Autodesk Inventor part; units mm, degrees
(part 2 of 2)
sketch "Sketch6" plane through (-21, -26.6, 14.3) normal (0, -1, 0) x (1, 0, 0)
  circle A0 centre (20, -9.6433) radius 3 projected
  arc A1 (9.5506, -10.6725) -> (10.7134, -10.9278) centre (11.3219, -5.3807) ccw projected
  arc A2 (10.7134, -10.9278) -> (10.771, -11.2914) centre (20, -9.6433) ccw projected
  arc A3 (10.771, -11.2914) -> (9.744, -11.8936) centre (13.0638, -16.379) ccw projected
  arc A4 (9.744, -11.8936) -> (9.8402, -12.2945) centre (20, -9.6433) ccw projected
  arc A5 (9.8402, -12.2945) -> (11.0287, -12.3648) centre (10.7619, -6.7907) ccw projected
  arc A6 (11.0287, -12.3648) -> (11.1424, -12.7149) centre (20, -9.6433) ccw projected
  arc A7 (11.1424, -12.7149) -> (10.2222, -13.4703) centre (14.2029, -17.3812) ccw projected
  arc A8 (10.2222, -13.4703) -> (10.38, -13.8512) centre (20, -9.6433) ccw projected
  arc A9 (10.38, -13.8512) -> (11.5649, -13.7347) centre (10.4294, -8.271) ccw projected
  arc A10 (11.5649, -13.7347) -> (11.732, -14.0627) centre (20, -9.6433) ccw projected
  arc A11 (11.732, -14.0627) -> (10.9413, -14.9527) centre (15.4848, -18.1928) ccw projected
  arc A12 (10.9413, -14.9527) -> (11.1567, -15.3043) centre (20, -9.6433) ccw projected
  arc A13 (11.1567, -15.3043) -> (12.3087, -15.0039) centre (10.3325, -9.7851) ccw projected
  arc A14 (12.3087, -15.0039) -> (12.5251, -15.3017) centre (20, -9.6433) ccw projected
  arc A15 (12.5251, -15.3017) -> (11.8834, -16.3045) centre (16.8778, -18.7939) ccw projected
  arc A16 (11.8834, -16.3045) -> (12.1512, -16.618) centre (20, -9.6433) ccw projected
  arc A17 (12.1512, -16.618) -> (13.242, -16.141) centre (10.4737, -11.2957) ccw projected
  arc A18 (13.242, -16.141) -> (13.5023, -16.4013) centre (20, -9.6433) ccw projected
  arc A19 (13.5023, -16.4013) -> (13.0253, -17.4922) centre (18.3477, -19.1696) ccw projected
  arc A20 (13.0253, -17.4922) -> (13.3389, -17.7599) centre (20, -9.6433) ccw projected
  arc A21 (13.3389, -17.7599) -> (14.3417, -17.1182) centre (10.8495, -12.7656) ccw projected
  arc A22 (14.3417, -17.1182) -> (14.6395, -17.3346) centre (20, -9.6433) ccw projected
  arc A23 (14.6395, -17.3346) -> (14.339, -18.4866) centre (19.8582, -19.3108) ccw projected
  arc A24 (14.339, -18.4866) -> (14.6906, -18.7021) centre (20, -9.6433) ccw projected
  arc A25 (14.6906, -18.7021) -> (15.5807, -17.9114) centre (11.4506, -14.1586) ccw projected
  arc A26 (15.5807, -17.9114) -> (15.9087, -18.0785) centre (20, -9.6433) ccw projected
  arc A27 (15.9087, -18.0785) -> (15.7921, -19.2633) centre (21.3723, -19.214) ccw projected
  arc A28 (15.7921, -19.2633) -> (16.1731, -19.4211) centre (20, -9.6433) ccw projected
  arc A29 (16.1731, -19.4211) -> (16.9285, -18.5009) centre (12.2622, -15.4404) ccw projected
  arc A30 (16.9285, -18.5009) -> (17.2786, -18.6147) centre (20, -9.6433) ccw projected
  arc A31 (17.2786, -18.6147) -> (17.3488, -19.8031) centre (22.8526, -18.8815) ccw projected
  arc A32 (17.3488, -19.8031) -> (17.7498, -19.8994) centre (20, -9.6433) ccw projected
  arc A33 (17.7498, -19.8994) -> (18.3519, -18.8723) centre (13.2643, -16.5795) ccw projected
  arc A34 (18.3519, -18.8723) -> (18.7155, -18.9299) centre (20, -9.6433) ccw projected
  arc A35 (18.7155, -18.9299) -> (18.9708, -20.0928) centre (24.2626, -18.3215) ccw projected
  arc A36 (18.9708, -20.0928) -> (19.3819, -20.1251) centre (20, -9.6433) ccw projected
  arc A37 (19.3819, -20.1251) -> (19.8159, -19.0165) centre (14.4323, -17.5478) ccw projected
  arc A38 (19.8159, -19.0165) -> (20.1841, -19.0165) centre (20, -9.6433) ccw projected
  arc A39 (20.1841, -19.0165) -> (20.6181, -20.1251) centre (25.5677, -17.5478) ccw projected
  arc A40 (20.6181, -20.1251) -> (21.0292, -20.0928) centre (20, -9.6433) ccw projected
  arc A41 (21.0292, -20.0928) -> (21.2845, -18.9299) centre (15.7374, -18.3215) ccw projected
  arc A42 (21.2845, -18.9299) -> (21.6481, -18.8723) centre (20, -9.6433) ccw projected
  arc A43 (21.6481, -18.8723) -> (22.2502, -19.8994) centre (26.7357, -16.5795) ccw projected
  arc A44 (22.2502, -19.8994) -> (22.6512, -19.8031) centre (20, -9.6433) ccw projected
  arc A45 (22.6512, -19.8031) -> (22.7214, -18.6147) centre (17.1474, -18.8815) ccw projected
  arc A46 (22.7214, -18.6147) -> (23.0715, -18.5009) centre (20, -9.6433) ccw projected
  arc A47 (23.0715, -18.5009) -> (23.8269, -19.4211) centre (27.7378, -15.4404) ccw projected
  arc A48 (23.8269, -19.4211) -> (24.2079, -19.2633) centre (20, -9.6433) ccw projected
  arc A49 (24.2079, -19.2633) -> (24.0913, -18.0785) centre (18.6277, -19.214) ccw projected
  arc A50 (24.0913, -18.0785) -> (24.4193, -17.9114) centre (20, -9.6433) ccw projected
  arc A51 (24.4193, -17.9114) -> (25.3094, -18.7021) centre (28.5494, -14.1586) ccw projected
  arc A52 (25.3094, -18.7021) -> (25.661, -18.4866) centre (20, -9.6433) ccw projected
  arc A53 (25.661, -18.4866) -> (25.3605, -17.3346) centre (20.1418, -19.3108) ccw projected
  arc A54 (25.3605, -17.3346) -> (25.6583, -17.1182) centre (20, -9.6433) ccw projected
  arc A55 (25.6583, -17.1182) -> (26.6611, -17.7599) centre (29.1505, -12.7656) ccw projected
  arc A56 (26.6611, -17.7599) -> (26.9747, -17.4922) centre (20, -9.6433) ccw projected
  arc A57 (26.9747, -17.4922) -> (26.4977, -16.4013) centre (21.6523, -19.1696) ccw projected
  arc A58 (26.4977, -16.4013) -> (26.758, -16.141) centre (20, -9.6433) ccw projected
  arc A59 (26.758, -16.141) -> (27.8488, -16.618) centre (29.5263, -11.2957) ccw projected
  arc A60 (27.8488, -16.618) -> (28.1166, -16.3045) centre (20, -9.6433) ccw projected
  arc A61 (28.1166, -16.3045) -> (27.4749, -15.3017) centre (23.1222, -18.7939) ccw projected
  arc A62 (27.4749, -15.3017) -> (27.6913, -15.0039) centre (20, -9.6433) ccw projected
  arc A63 (27.6913, -15.0039) -> (28.8433, -15.3043) centre (29.6675, -9.7851) ccw projected
  arc A64 (28.8433, -15.3043) -> (29.0587, -14.9527) centre (20, -9.6433) ccw projected
  arc A65 (29.0587, -14.9527) -> (28.268, -14.0627) centre (24.5152, -18.1928) ccw projected
  arc A66 (28.268, -14.0627) -> (28.4351, -13.7347) centre (20, -9.6433) ccw projected
  arc A67 (28.4351, -13.7347) -> (29.62, -13.8512) centre (29.5706, -8.271) ccw projected
  arc A68 (29.62, -13.8512) -> (29.7778, -13.4703) centre (20, -9.6433) ccw projected
  arc A69 (29.7778, -13.4703) -> (28.8576, -12.7149) centre (25.7971, -17.3812) ccw projected
  arc A70 (28.8576, -12.7149) -> (28.9713, -12.3648) centre (20, -9.6433) ccw projected
  arc A71 (28.9713, -12.3648) -> (30.1598, -12.2945) centre (29.2381, -6.7907) ccw projected
  arc A72 (30.1598, -12.2945) -> (30.256, -11.8936) centre (20, -9.6433) ccw projected
  arc A73 (30.256, -11.8936) -> (29.229, -11.2914) centre (26.9362, -16.379) ccw projected
  arc A74 (29.229, -11.2914) -> (29.2866, -10.9278) centre (20, -9.6433) ccw projected
  arc A75 (29.2866, -10.9278) -> (30.4494, -10.6725) centre (28.6781, -5.3807) ccw projected
  arc A76 (30.4494, -10.6725) -> (30.4818, -10.2615) centre (20, -9.6433) ccw projected
  arc A77 (30.4818, -10.2615) -> (29.3732, -9.8274) centre (27.9045, -15.2111) ccw projected
  arc A78 (29.3732, -9.8274) -> (29.3732, -9.4593) centre (20, -9.6433) ccw projected
  arc A79 (29.3732, -9.4593) -> (30.4818, -9.0252) centre (27.9045, -4.0756) ccw projected
  arc A80 (30.4818, -9.0252) -> (30.4494, -8.6142) centre (20, -9.6433) ccw projected
  arc A81 (30.4494, -8.6142) -> (29.2866, -8.3588) centre (28.6781, -13.906) ccw projected
  arc A82 (29.2866, -8.3588) -> (29.229, -7.9952) centre (20, -9.6433) ccw projected
  arc A83 (29.229, -7.9952) -> (30.256, -7.3931) centre (26.9362, -2.9076) ccw projected
  arc A84 (30.256, -7.3931) -> (30.1598, -6.9922) centre (20, -9.6433) ccw projected
  arc A85 (30.1598, -6.9922) -> (28.9713, -6.9219) centre (29.2381, -12.4959) ccw projected
  arc A86 (28.9713, -6.9219) -> (28.8576, -6.5718) centre (20, -9.6433) ccw projected
  arc A87 (28.8576, -6.5718) -> (29.7778, -5.8164) centre (25.7971, -1.9055) ccw projected
  arc A88 (29.7778, -5.8164) -> (29.62, -5.4355) centre (20, -9.6433) ccw projected
  arc A89 (29.62, -5.4355) -> (28.4351, -5.552) centre (29.5706, -11.0157) ccw projected
  arc A90 (28.4351, -5.552) -> (28.268, -5.224) centre (20, -9.6433) ccw projected
  arc A91 (28.268, -5.224) -> (29.0587, -4.3339) centre (24.5152, -1.0939) ccw projected
  arc A92 (29.0587, -4.3339) -> (28.8433, -3.9824) centre (20, -9.6433) ccw projected
  arc A93 (28.8433, -3.9824) -> (27.6913, -4.2828) centre (29.6675, -9.5016) ccw projected
  arc A94 (27.6913, -4.2828) -> (27.4749, -3.985) centre (20, -9.6433) ccw projected
  arc A95 (27.4749, -3.985) -> (28.1166, -2.9822) centre (23.1222, -0.4928) ccw projected
  arc A96 (28.1166, -2.9822) -> (27.8488, -2.6687) centre (20, -9.6433) ccw projected
  arc A97 (27.8488, -2.6687) -> (26.758, -3.1456) centre (29.5263, -7.991) ccw projected
  arc A98 (26.758, -3.1456) -> (26.4977, -2.8853) centre (20, -9.6433) ccw projected
  arc A99 (26.4977, -2.8853) -> (26.9747, -1.7945) centre (21.6523, -0.1171) ccw projected
  arc A100 (26.9747, -1.7945) -> (26.6611, -1.5267) centre (20, -9.6433) ccw projected
  arc A101 (26.6611, -1.5267) -> (25.6583, -2.1685) centre (29.1505, -6.5211) ccw projected
  arc A102 (25.6583, -2.1685) -> (25.3605, -1.9521) centre (20, -9.6433) ccw projected
  arc A103 (25.3605, -1.9521) -> (25.661, -0.8001) centre (20.1418, 0.0241) ccw projected
  arc A104 (25.661, -0.8001) -> (25.3094, -0.5846) centre (20, -9.6433) ccw projected
  arc A105 (25.3094, -0.5846) -> (24.4193, -1.3753) centre (28.5494, -5.1281) ccw projected
  arc A106 (24.4193, -1.3753) -> (24.0913, -1.2082) centre (20, -9.6433) ccw projected
  arc A107 (24.0913, -1.2082) -> (24.2079, -0.0234) centre (18.6277, -0.0727) ccw projected
  arc A108 (24.2079, -0.0234) -> (23.8269, 0.1344) centre (20, -9.6433) ccw projected
  arc A109 (23.8269, 0.1344) -> (23.0715, -0.7858) centre (27.7378, -3.8463) ccw projected
  arc A110 (23.0715, -0.7858) -> (22.7214, -0.672) centre (20, -9.6433) ccw projected
  arc A111 (22.7214, -0.672) -> (22.6512, 0.5165) centre (17.1474, -0.4052) ccw projected
  arc A112 (22.6512, 0.5165) -> (22.2502, 0.6127) centre (20, -9.6433) ccw projected
  arc A113 (22.2502, 0.6127) -> (21.6481, -0.4143) centre (26.7357, -2.7072) ccw projected
  arc A114 (21.6481, -0.4143) -> (21.2845, -0.3568) centre (20, -9.6433) ccw projected
  arc A115 (21.2845, -0.3568) -> (21.0292, 0.8061) centre (15.7374, -0.9652) ccw projected
  arc A116 (21.0292, 0.8061) -> (20.6181, 0.8384) centre (20, -9.6433) ccw projected
  arc A117 (20.6181, 0.8384) -> (20.1841, -0.2701) centre (25.5677, -1.7389) ccw projected
  arc A118 (20.1841, -0.2701) -> (19.8159, -0.2701) centre (20, -9.6433) ccw projected
  arc A119 (19.8159, -0.2701) -> (19.3819, 0.8384) centre (14.4323, -1.7389) ccw projected
  arc A120 (19.3819, 0.8384) -> (18.9708, 0.8061) centre (20, -9.6433) ccw projected
  arc A121 (18.9708, 0.8061) -> (18.7155, -0.3568) centre (24.2626, -0.9652) ccw projected
  arc A122 (18.7155, -0.3568) -> (18.3519, -0.4143) centre (20, -9.6433) ccw projected
  arc A123 (18.3519, -0.4143) -> (17.7498, 0.6127) centre (13.2643, -2.7072) ccw projected
  arc A124 (17.7498, 0.6127) -> (17.3488, 0.5165) centre (20, -9.6433) ccw projected
  arc A125 (17.3488, 0.5165) -> (17.2786, -0.672) centre (22.8526, -0.4052) ccw projected
  arc A126 (17.2786, -0.672) -> (16.9285, -0.7858) centre (20, -9.6433) ccw projected
  arc A127 (16.9285, -0.7858) -> (16.1731, 0.1344) centre (12.2622, -3.8463) ccw projected
  arc A128 (16.1731, 0.1344) -> (15.7921, -0.0234) centre (20, -9.6433) ccw projected
  arc A129 (15.7921, -0.0234) -> (15.9087, -1.2082) centre (21.3723, -0.0727) ccw projected
  arc A130 (15.9087, -1.2082) -> (15.5807, -1.3753) centre (20, -9.6433) ccw projected
  arc A131 (15.5807, -1.3753) -> (14.6906, -0.5846) centre (11.4506, -5.1281) ccw projected
  arc A132 (14.6906, -0.5846) -> (14.339, -0.8001) centre (20, -9.6433) ccw projected
  arc A133 (14.339, -0.8001) -> (14.6395, -1.9521) centre (19.8582, 0.0241) ccw projected
  arc A134 (14.6395, -1.9521) -> (14.3417, -2.1685) centre (20, -9.6433) ccw projected
  arc A135 (14.3417, -2.1685) -> (13.3389, -1.5267) centre (10.8495, -6.5211) ccw projected
  arc A136 (13.3389, -1.5267) -> (13.0253, -1.7945) centre (20, -9.6433) ccw projected
  arc A137 (13.0253, -1.7945) -> (13.5023, -2.8853) centre (18.3477, -0.1171) ccw projected
  arc A138 (13.5023, -2.8853) -> (13.242, -3.1456) centre (20, -9.6433) ccw projected
  arc A139 (13.242, -3.1456) -> (12.1512, -2.6687) centre (10.4737, -7.991) ccw projected
  arc A140 (12.1512, -2.6687) -> (11.8834, -2.9822) centre (20, -9.6433) ccw projected
  arc A141 (11.8834, -2.9822) -> (12.5251, -3.985) centre (16.8778, -0.4928) ccw projected
  arc A142 (12.5251, -3.985) -> (12.3087, -4.2828) centre (20, -9.6433) ccw projected
  arc A143 (12.3087, -4.2828) -> (11.1567, -3.9824) centre (10.3325, -9.5016) ccw projected
  arc A144 (11.1567, -3.9824) -> (10.9413, -4.3339) centre (20, -9.6433) ccw projected
  arc A145 (10.9413, -4.3339) -> (11.732, -5.224) centre (15.4848, -1.0939) ccw projected
  arc A146 (11.732, -5.224) -> (11.5649, -5.552) centre (20, -9.6433) ccw projected
  arc A147 (11.5649, -5.552) -> (10.38, -5.4355) centre (10.4294, -11.0157) ccw projected
  arc A148 (10.38, -5.4355) -> (10.2222, -5.8164) centre (20, -9.6433) ccw projected
  arc A149 (10.2222, -5.8164) -> (11.1424, -6.5718) centre (14.2029, -1.9055) ccw projected
  arc A150 (11.1424, -6.5718) -> (11.0287, -6.9219) centre (20, -9.6433) ccw projected
  arc A151 (11.0287, -6.9219) -> (9.8402, -6.9922) centre (10.7619, -12.4959) ccw projected
  arc A152 (9.8402, -6.9922) -> (9.744, -7.3931) centre (20, -9.6433) ccw projected
  arc A153 (9.744, -7.3931) -> (10.771, -7.9952) centre (13.0638, -2.9076) ccw projected
  arc A154 (10.771, -7.9952) -> (10.7134, -8.3588) centre (20, -9.6433) ccw projected
  arc A155 (10.7134, -8.3588) -> (9.5506, -8.6142) centre (11.3219, -13.906) ccw projected
  arc A156 (9.5506, -8.6142) -> (9.5182, -9.0252) centre (20, -9.6433) ccw projected
  arc A157 (9.5182, -9.0252) -> (10.6268, -9.4593) centre (12.0955, -4.0756) ccw projected
  arc A158 (10.6268, -9.4593) -> (10.6268, -9.8274) centre (20, -9.6433) ccw projected
  arc A159 (10.6268, -9.8274) -> (9.5182, -10.2615) centre (12.0955, -15.2111) ccw projected
  arc A160 (9.5182, -10.2615) -> (9.5506, -10.6725) centre (20, -9.6433) ccw projected
  circle A161 centre (47, -9.6433) radius 3 projected
  arc A162 (57.4494, -8.6142) -> (56.2866, -8.3588) centre (55.6781, -13.906) ccw projected
  arc A163 (56.2866, -8.3588) -> (56.229, -7.9952) centre (47, -9.6433) ccw projected
  arc A164 (56.229, -7.9952) -> (57.256, -7.3931) centre (53.9362, -2.9076) ccw projected
  arc A165 (57.256, -7.3931) -> (57.1598, -6.9922) centre (47, -9.6433) ccw projected
  arc A166 (57.1598, -6.9922) -> (55.9713, -6.9219) centre (56.2381, -12.4959) ccw projected
  arc A167 (55.9713, -6.9219) -> (55.8576, -6.5718) centre (47, -9.6433) ccw projected
  arc A168 (55.8576, -6.5718) -> (56.7778, -5.8164) centre (52.7971, -1.9055) ccw projected
  arc A169 (56.7778, -5.8164) -> (56.62, -5.4355) centre (47, -9.6433) ccw projected
  arc A170 (56.62, -5.4355) -> (55.4351, -5.552) centre (56.5706, -11.0157) ccw projected
  arc A171 (55.4351, -5.552) -> (55.268, -5.224) centre (47, -9.6433) ccw projected
  arc A172 (55.268, -5.224) -> (56.0587, -4.3339) centre (51.5152, -1.0939) ccw projected
  arc A173 (56.0587, -4.3339) -> (55.8433, -3.9824) centre (47, -9.6433) ccw projected
  arc A174 (55.8433, -3.9824) -> (54.6913, -4.2828) centre (56.6675, -9.5016) ccw projected
  arc A175 (54.6913, -4.2828) -> (54.4749, -3.985) centre (47, -9.6433) ccw projected
  arc A176 (54.4749, -3.985) -> (55.1166, -2.9822) centre (50.1222, -0.4928) ccw projected
  arc A177 (55.1166, -2.9822) -> (54.8488, -2.6687) centre (47, -9.6433) ccw projected
  arc A178 (54.8488, -2.6687) -> (53.758, -3.1456) centre (56.5263, -7.991) ccw projected
  arc A179 (53.758, -3.1456) -> (53.4977, -2.8853) centre (47, -9.6433) ccw projected
  arc A180 (53.4977, -2.8853) -> (53.9747, -1.7945) centre (48.6523, -0.1171) ccw projected
  arc A181 (53.9747, -1.7945) -> (53.6611, -1.5267) centre (47, -9.6433) ccw projected
  arc A182 (53.6611, -1.5267) -> (52.6583, -2.1685) centre (56.1505, -6.5211) ccw projected
  arc A183 (52.6583, -2.1685) -> (52.3605, -1.9521) centre (47, -9.6433) ccw projected
  arc A184 (52.3605, -1.9521) -> (52.661, -0.8001) centre (47.1418, 0.0241) ccw projected
  arc A185 (52.661, -0.8001) -> (52.3094, -0.5846) centre (47, -9.6433) ccw projected
  arc A186 (52.3094, -0.5846) -> (51.4193, -1.3753) centre (55.5494, -5.1281) ccw projected
  arc A187 (51.4193, -1.3753) -> (51.0913, -1.2082) centre (47, -9.6433) ccw projected
  arc A188 (51.0913, -1.2082) -> (51.2079, -0.0234) centre (45.6277, -0.0727) ccw projected
  arc A189 (51.2079, -0.0234) -> (50.8269, 0.1344) centre (47, -9.6433) ccw projected
  arc A190 (50.8269, 0.1344) -> (50.0715, -0.7858) centre (54.7378, -3.8463) ccw projected
  arc A191 (50.0715, -0.7858) -> (49.7214, -0.672) centre (47, -9.6433) ccw projected
  arc A192 (49.7214, -0.672) -> (49.6512, 0.5165) centre (44.1474, -0.4052) ccw projected
  arc A193 (49.6512, 0.5165) -> (49.2502, 0.6127) centre (47, -9.6433) ccw projected
  arc A194 (49.2502, 0.6127) -> (48.6481, -0.4143) centre (53.7357, -2.7072) ccw projected
  arc A195 (48.6481, -0.4143) -> (48.2845, -0.3568) centre (47, -9.6433) ccw projected
  arc A196 (48.2845, -0.3568) -> (48.0292, 0.8061) centre (42.7374, -0.9652) ccw projected
  arc A197 (48.0292, 0.8061) -> (47.6181, 0.8384) centre (47, -9.6433) ccw projected
  arc A198 (47.6181, 0.8384) -> (47.1841, -0.2701) centre (52.5677, -1.7389) ccw projected
  arc A199 (47.1841, -0.2701) -> (46.8159, -0.2701) centre (47, -9.6433) ccw projected
  arc A200 (46.8159, -0.2701) -> (46.3819, 0.8384) centre (41.4323, -1.7389) ccw projected
  arc A201 (46.3819, 0.8384) -> (45.9708, 0.8061) centre (47, -9.6433) ccw projected
  arc A202 (45.9708, 0.8061) -> (45.7155, -0.3568) centre (51.2626, -0.9652) ccw projected
  arc A203 (45.7155, -0.3568) -> (45.3519, -0.4143) centre (47, -9.6433) ccw projected
  arc A204 (45.3519, -0.4143) -> (44.7498, 0.6127) centre (40.2643, -2.7072) ccw projected
  arc A205 (44.7498, 0.6127) -> (44.3488, 0.5165) centre (47, -9.6433) ccw projected
  arc A206 (44.3488, 0.5165) -> (44.2786, -0.672) centre (49.8526, -0.4052) ccw projected
  arc A207 (44.2786, -0.672) -> (43.9285, -0.7858) centre (47, -9.6433) ccw projected
  arc A208 (43.9285, -0.7858) -> (43.1731, 0.1344) centre (39.2622, -3.8463) ccw projected
  arc A209 (43.1731, 0.1344) -> (42.7921, -0.0234) centre (47, -9.6433) ccw projected
  arc A210 (42.7921, -0.0234) -> (42.9087, -1.2082) centre (48.3723, -0.0727) ccw projected
  arc A211 (42.9087, -1.2082) -> (42.5807, -1.3753) centre (47, -9.6433) ccw projected
  arc A212 (42.5807, -1.3753) -> (41.6906, -0.5846) centre (38.4506, -5.1281) ccw projected
  arc A213 (41.6906, -0.5846) -> (41.339, -0.8001) centre (47, -9.6433) ccw projected
  arc A214 (41.339, -0.8001) -> (41.6395, -1.9521) centre (46.8582, 0.0241) ccw projected
  arc A215 (41.6395, -1.9521) -> (41.3417, -2.1685) centre (47, -9.6433) ccw projected
  arc A216 (41.3417, -2.1685) -> (40.3389, -1.5267) centre (37.8495, -6.5211) ccw projected
  arc A217 (40.3389, -1.5267) -> (40.0253, -1.7945) centre (47, -9.6433) ccw projected
  arc A218 (40.0253, -1.7945) -> (40.5023, -2.8853) centre (45.3477, -0.1171) ccw projected
  arc A219 (40.5023, -2.8853) -> (40.242, -3.1456) centre (47, -9.6433) ccw projected
  arc A220 (40.242, -3.1456) -> (39.1512, -2.6687) centre (37.4737, -7.991) ccw projected
  arc A221 (39.1512, -2.6687) -> (38.8834, -2.9822) centre (47, -9.6433) ccw projected
  arc A222 (38.8834, -2.9822) -> (39.5251, -3.985) centre (43.8778, -0.4928) ccw projected
  arc A223 (39.5251, -3.985) -> (39.3087, -4.2828) centre (47, -9.6433) ccw projected
  arc A224 (39.3087, -4.2828) -> (38.1567, -3.9824) centre (37.3325, -9.5016) ccw projected
  arc A225 (38.1567, -3.9824) -> (37.9413, -4.3339) centre (47, -9.6433) ccw projected
  arc A226 (37.9413, -4.3339) -> (38.732, -5.224) centre (42.4848, -1.0939) ccw projected
  arc A227 (38.732, -5.224) -> (38.5649, -5.552) centre (47, -9.6433) ccw projected
  arc A228 (38.5649, -5.552) -> (37.38, -5.4355) centre (37.4294, -11.0157) ccw projected
  arc A229 (37.38, -5.4355) -> (37.2222, -5.8164) centre (47, -9.6433) ccw projected
  arc A230 (37.2222, -5.8164) -> (38.1424, -6.5718) centre (41.2029, -1.9055) ccw projected
  arc A231 (38.1424, -6.5718) -> (38.0287, -6.9219) centre (47, -9.6433) ccw projected
  arc A232 (38.0287, -6.9219) -> (36.8402, -6.9922) centre (37.7619, -12.4959) ccw projected
  arc A233 (36.8402, -6.9922) -> (36.744, -7.3931) centre (47, -9.6433) ccw projected
  arc A234 (36.744, -7.3931) -> (37.771, -7.9952) centre (40.0638, -2.9076) ccw projected
  arc A235 (37.771, -7.9952) -> (37.7134, -8.3588) centre (47, -9.6433) ccw projected
  arc A236 (37.7134, -8.3588) -> (36.5506, -8.6142) centre (38.3219, -13.906) ccw projected
  arc A237 (36.5506, -8.6142) -> (36.5182, -9.0252) centre (47, -9.6433) ccw projected
  arc A238 (36.5182, -9.0252) -> (37.6268, -9.4593) centre (39.0955, -4.0756) ccw projected
  arc A239 (37.6268, -9.4593) -> (37.6268, -9.8274) centre (47, -9.6433) ccw projected
  arc A240 (37.6268, -9.8274) -> (36.5182, -10.2615) centre (39.0955, -15.2111) ccw projected
  arc A241 (36.5182, -10.2615) -> (36.5506, -10.6725) centre (47, -9.6433) ccw projected
  arc A242 (36.5506, -10.6725) -> (37.7134, -10.9278) centre (38.3219, -5.3807) ccw projected
  arc A243 (37.7134, -10.9278) -> (37.771, -11.2914) centre (47, -9.6433) ccw projected
  arc A244 (37.771, -11.2914) -> (36.744, -11.8936) centre (40.0638, -16.379) ccw projected
  arc A245 (36.744, -11.8936) -> (36.8402, -12.2945) centre (47, -9.6433) ccw projected
  arc A246 (36.8402, -12.2945) -> (38.0287, -12.3648) centre (37.7619, -6.7907) ccw projected
  arc A247 (38.0287, -12.3648) -> (38.1424, -12.7149) centre (47, -9.6433) ccw projected
  arc A248 (38.1424, -12.7149) -> (37.2222, -13.4703) centre (41.2029, -17.3812) ccw projected
  arc A249 (37.2222, -13.4703) -> (37.38, -13.8512) centre (47, -9.6433) ccw projected
  arc A250 (37.38, -13.8512) -> (38.5649, -13.7347) centre (37.4294, -8.271) ccw projected
  arc A251 (38.5649, -13.7347) -> (38.732, -14.0627) centre (47, -9.6433) ccw projected
  arc A252 (38.732, -14.0627) -> (37.9413, -14.9527) centre (42.4848, -18.1928) ccw projected
  arc A253 (37.9413, -14.9527) -> (38.1567, -15.3043) centre (47, -9.6433) ccw projected
  arc A254 (38.1567, -15.3043) -> (39.3087, -15.0039) centre (37.3325, -9.7851) ccw projected
  arc A255 (39.3087, -15.0039) -> (39.5251, -15.3017) centre (47, -9.6433) ccw projected
  arc A256 (39.5251, -15.3017) -> (38.8834, -16.3045) centre (43.8778, -18.7939) ccw projected
  arc A257 (38.8834, -16.3045) -> (39.1512, -16.618) centre (47, -9.6433) ccw projected
  arc A258 (39.1512, -16.618) -> (40.242, -16.141) centre (37.4737, -11.2957) ccw projected
  arc A259 (40.242, -16.141) -> (40.5023, -16.4013) centre (47, -9.6433) ccw projected
  arc A260 (40.5023, -16.4013) -> (40.0253, -17.4922) centre (45.3477, -19.1696) ccw projected
  arc A261 (40.0253, -17.4922) -> (40.3389, -17.7599) centre (47, -9.6433) ccw projected
  arc A262 (40.3389, -17.7599) -> (41.3417, -17.1182) centre (37.8495, -12.7656) ccw projected
  arc A263 (41.3417, -17.1182) -> (41.6395, -17.3346) centre (47, -9.6433) ccw projected
  arc A264 (41.6395, -17.3346) -> (41.339, -18.4866) centre (46.8582, -19.3108) ccw projected
  arc A265 (41.339, -18.4866) -> (41.6906, -18.7021) centre (47, -9.6433) ccw projected
  arc A266 (41.6906, -18.7021) -> (42.5807, -17.9114) centre (38.4506, -14.1586) ccw projected
  arc A267 (42.5807, -17.9114) -> (42.9087, -18.0785) centre (47, -9.6433) ccw projected
  arc A268 (42.9087, -18.0785) -> (42.7921, -19.2633) centre (48.3723, -19.214) ccw projected
  arc A269 (42.7921, -19.2633) -> (43.1731, -19.4211) centre (47, -9.6433) ccw projected
  arc A270 (43.1731, -19.4211) -> (43.9285, -18.5009) centre (39.2622, -15.4404) ccw projected
  arc A271 (43.9285, -18.5009) -> (44.2786, -18.6147) centre (47, -9.6433) ccw projected
  arc A272 (44.2786, -18.6147) -> (44.3488, -19.8031) centre (49.8526, -18.8815) ccw projected
  arc A273 (44.3488, -19.8031) -> (44.7498, -19.8994) centre (47, -9.6433) ccw projected
  arc A274 (44.7498, -19.8994) -> (45.3519, -18.8723) centre (40.2643, -16.5795) ccw projected
  arc A275 (45.3519, -18.8723) -> (45.7155, -18.9299) centre (47, -9.6433) ccw projected
  arc A276 (45.7155, -18.9299) -> (45.9708, -20.0928) centre (51.2626, -18.3215) ccw projected
  arc A277 (45.9708, -20.0928) -> (46.3819, -20.1251) centre (47, -9.6433) ccw projected
  arc A278 (46.3819, -20.1251) -> (46.8159, -19.0165) centre (41.4323, -17.5478) ccw projected
  arc A279 (46.8159, -19.0165) -> (47.1841, -19.0165) centre (47, -9.6433) ccw projected
  arc A280 (47.1841, -19.0165) -> (47.6181, -20.1251) centre (52.5677, -17.5478) ccw projected
  arc A281 (47.6181, -20.1251) -> (48.0292, -20.0928) centre (47, -9.6433) ccw projected
  arc A282 (48.0292, -20.0928) -> (48.2845, -18.9299) centre (42.7374, -18.3215) ccw projected
  arc A283 (48.2845, -18.9299) -> (48.6481, -18.8723) centre (47, -9.6433) ccw projected
  arc A284 (48.6481, -18.8723) -> (49.2502, -19.8994) centre (53.7357, -16.5795) ccw projected
  arc A285 (49.2502, -19.8994) -> (49.6512, -19.8031) centre (47, -9.6433) ccw projected
  arc A286 (49.6512, -19.8031) -> (49.7214, -18.6147) centre (44.1474, -18.8815) ccw projected
  arc A287 (49.7214, -18.6147) -> (50.0715, -18.5009) centre (47, -9.6433) ccw projected
  arc A288 (50.0715, -18.5009) -> (50.8269, -19.4211) centre (54.7378, -15.4404) ccw projected
  arc A289 (50.8269, -19.4211) -> (51.2079, -19.2633) centre (47, -9.6433) ccw projected
  arc A290 (51.2079, -19.2633) -> (51.0913, -18.0785) centre (45.6277, -19.214) ccw projected
  arc A291 (51.0913, -18.0785) -> (51.4193, -17.9114) centre (47, -9.6433) ccw projected
  arc A292 (51.4193, -17.9114) -> (52.3094, -18.7021) centre (55.5494, -14.1586) ccw projected
  arc A293 (52.3094, -18.7021) -> (52.661, -18.4866) centre (47, -9.6433) ccw projected
  arc A294 (52.661, -18.4866) -> (52.3605, -17.3346) centre (47.1418, -19.3108) ccw projected
  arc A295 (52.3605, -17.3346) -> (52.6583, -17.1182) centre (47, -9.6433) ccw projected
  arc A296 (52.6583, -17.1182) -> (53.6611, -17.7599) centre (56.1505, -12.7656) ccw projected
  arc A297 (53.6611, -17.7599) -> (53.9747, -17.4922) centre (47, -9.6433) ccw projected
  arc A298 (53.9747, -17.4922) -> (53.4977, -16.4013) centre (48.6523, -19.1696) ccw projected
  arc A299 (53.4977, -16.4013) -> (53.758, -16.141) centre (47, -9.6433) ccw projected
  arc A300 (53.758, -16.141) -> (54.8488, -16.618) centre (56.5263, -11.2957) ccw projected
  arc A301 (54.8488, -16.618) -> (55.1166, -16.3045) centre (47, -9.6433) ccw projected
  arc A302 (55.1166, -16.3045) -> (54.4749, -15.3017) centre (50.1222, -18.7939) ccw projected
  arc A303 (54.4749, -15.3017) -> (54.6913, -15.0039) centre (47, -9.6433) ccw projected
  arc A304 (54.6913, -15.0039) -> (55.8433, -15.3043) centre (56.6675, -9.7851) ccw projected
  arc A305 (55.8433, -15.3043) -> (56.0587, -14.9527) centre (47, -9.6433) ccw projected
  arc A306 (56.0587, -14.9527) -> (55.268, -14.0627) centre (51.5152, -18.1928) ccw projected
  arc A307 (55.268, -14.0627) -> (55.4351, -13.7347) centre (47, -9.6433) ccw projected
  arc A308 (55.4351, -13.7347) -> (56.62, -13.8512) centre (56.5706, -8.271) ccw projected
  arc A309 (56.62, -13.8512) -> (56.7778, -13.4703) centre (47, -9.6433) ccw projected
  arc A310 (56.7778, -13.4703) -> (55.8576, -12.7149) centre (52.7971, -17.3812) ccw projected
  arc A311 (55.8576, -12.7149) -> (55.9713, -12.3648) centre (47, -9.6433) ccw projected
  arc A312 (55.9713, -12.3648) -> (57.1598, -12.2945) centre (56.2381, -6.7907) ccw projected
  arc A313 (57.1598, -12.2945) -> (57.256, -11.8936) centre (47, -9.6433) ccw projected
  arc A314 (57.256, -11.8936) -> (56.229, -11.2914) centre (53.9362, -16.379) ccw projected
  arc A315 (56.229, -11.2914) -> (56.2866, -10.9278) centre (47, -9.6433) ccw projected
  arc A316 (56.2866, -10.9278) -> (57.4494, -10.6725) centre (55.6781, -5.3807) ccw projected
  arc A317 (57.4494, -10.6725) -> (57.4818, -10.2615) centre (47, -9.6433) ccw projected
  arc A318 (57.4818, -10.2615) -> (56.3732, -9.8274) centre (54.9045, -15.2111) ccw projected
  arc A319 (56.3732, -9.8274) -> (56.3732, -9.4593) centre (47, -9.6433) ccw projected
  arc A320 (56.3732, -9.4593) -> (57.4818, -9.0252) centre (54.9045, -4.0756) ccw projected
  arc A321 (57.4818, -9.0252) -> (57.4494, -8.6142) centre (47, -9.6433) ccw projected
  circle A322 centre (20, -9.6433) radius 10.5
  circle A323 centre (47, -9.6433) radius 10.5
  circle A324 centre (20, -9.6433) radius 10.9
  circle A325 centre (47, -9.6433) radius 10.9
  arc A326 (29.092, 0.1172) -> (29.2864, -14.3) centre (33.5, -7.0333) ccw projected
  line L0 (6.5, -14.3) -> (29.2864, -14.3) projected
  arc A327 (36.2919, 9.8389) -> (29.092, 0.1172) centre (35.7557, 2.709) ccw projected
  arc A328 (49.3884, 4.2041) -> (36.2919, 9.8389) centre (43.0585, 7.5289) ccw projected
  arc A329 (41.3938, -1.688) -> (49.3884, 4.2041) centre (46.65, -0.45) ccw projected
  arc A330 (40.6022, -2.5478) -> (41.3938, -1.688) centre (35.7557, 2.709) ccw projected
  arc A331 (37.7136, -14.3) -> (40.6022, -2.5478) centre (33.5, -7.0333) ccw projected
  line L1 (37.7136, -14.3) -> (60.5, -14.3) projected
  line L2 (60.5, -14.3) -> (60.5, 13.4) projected
  line L3 (60.5, 13.4) -> (48.1174, 13.4) projected
  arc A332 (48.1174, 13.4) -> (37.9995, 13.4) centre (43.0585, 7.5289) ccw projected
  line L4 (37.9995, 13.4) -> (6.5, 13.4) projected
  line L5 (6.5, 13.4) -> (6.5, -14.3) projected
  point P0 (21, -14.3)
  point P1 (27.2086, -1.4674)
  point P2 (37.2633, -14.5431)
  point P3 (52.0289, 0.0273)
  point P4 (56.8552, -14.3)
  point P5 (10.1448, -14.3)
  dimension "d29" = 0.4
  dimension "d30" = 0.4
  constraints: 2 centre point, 2 coincident, 6 other
ref_plane "Work Plane4" through (-12.2915, -29.7, -6.6348) normal (0, -1, 0) x (0.9969173, 0, -0.0784591)
extrude "Extrusion6" add sketch "Sketch6" along normal blind 3.2 contours L0 L5 L4 A332 L3 L2 L1 A325 A329 A328 A327 A326 A324
sketch "Sketch7" plane through (-21, -26.6, 14.3) normal (0, -1, 0) x (1, 0, 0)
  circle A0 centre (47, -9.6433) radius 5.5 projected
  circle A1 centre (20, -9.6433) radius 5.5 projected
  circle A2 centre (20, -9.6433) radius 5.8
  circle A3 centre (47, -9.6433) radius 5.8
  point P0 (21, -14.3)
  dimension "d38" = 0.3
  dimension "d39" = 0.3
  constraints: 2 centre point
  measures "d38" radial gap between concentric circles of A1 A2
  measures "d39" radial gap between concentric circles of A0 A3
extrude "Extrusion7" cut sketch "Sketch7" against normal blind 1 contours A0 | A1 | A2 | A3
sketch "Sketch8" plane through (-21, -25.6, 14.3) normal (0, -1, 0) x (1, 0, 0)
  circle A0 centre (20, -9.6433) radius 4 projected
  circle A1 centre (47, -9.6433) radius 4 projected
  circle A2 centre (20, -9.6433) radius 4.3
  circle A3 centre (47, -9.6433) radius 4.3
  point P0 (21, -14.3)
  dimension "d42" = 0.3
  dimension "d43" = 0.3
  constraints: 2 centre point
  measures "d42" radial gap between concentric circles of A0 A2
  measures "d43" radial gap between concentric circles of A1 A3
extrude "Extrusion8" cut sketch "Sketch8" against normal through all contours A0 | A2
sketch "Sketch9" plane through (-21, -25.6, 14.3) normal (0, -1, 0) x (1, 0, 0)
  circle A0 centre (47, -9.6433) radius 4 projected
  circle A1 centre (47, -9.6433) radius 4.3
  point P0 (21, -14.3)
  dimension "d46" = 0.3
  constraints: 1 centre point
  measures "d46" radial gap between concentric circles of A0 A1
extrude "Extrusion9" cut sketch "Sketch9" against normal blind 7.2 contours A0 | A1
sketch "Sketch10" plane through (-21, -19.3, 14.3) normal (0, -1, 0) x (1, 0, 0)
  arc A0 (49.3884, 4.2041) -> (41.3503, 0.586) centre (46.65, -0.45) ccw projected
  circle A1 centre (43.0585, 7.5289) radius 7.15
  arc A2 (49.3884, 4.2041) -> (41.3503, 0.586) centre (43.0585, 7.5289) ccw projected
  point P0 (21, -14.3)
  point P1 (46.7585, 1.4108)
  point P2 (41.3503, 0.586)
  point P3 (49.3884, 4.2041)
  dimension "d145" = 0
  constraints: 1 coincident, 3 other
extrude "Extrusion10" cut sketch "Sketch10" against normal blind 0.1
sketch "Sketch11" plane through (-21, -19.2, 14.3) normal (0, -1, 0) x (1, 0, 0)
  circle A0 centre (43.0585, 7.5289) radius 1.25 projected
  circle A1 centre (43.0585, 7.5289) radius 3.45
  circle A2 centre (43.0585, 7.5289) radius 3.65
  point P0 (21, -14.3)
  dimension "d51" = 6.9
  dimension "d52" = 0.2
  constraints: 2 centre point, 1 coincident
  measures "d51" diameter of A1
  measures "d52" radial gap between concentric circles of A1 A2
extrude "Extrusion11" cut sketch "Sketch11" against normal blind 0.4 contours A0 | A1 | A2
sketch "Sketch12" plane through (39.5, -16.2, 0) normal (0, 0, -1) x (-1, 0, 0)
  line L0 (35.3905, 0) -> (35.3905, -5.3) projected
  line L1 (0, 0) -> (35.3905, 0) projected
  line L2 (0, 0) -> (0, -13.6) projected
  circle A0 centre (3.5, -3.5) radius 3.5
  line L3 (35.3905, -5.3) -> (27.3, -5.3) projected
  circle A1 centre (24.2983, -3.5) radius 3.5
  line L4 (45.8, -5.3) -> (35.3905, -5.3) projected
  line L5 (45.8, -5.3) -> (45.8, -8.3) projected
  line L6 (31.2136, -8.3) -> (22.7864, -8.3) projected
  line L7 (22.7864, -10.4) -> (16.9577, -10.4) projected
  line L8 (22.7864, -8.3) -> (22.7864, -10.4) projected
  line L9 (31.2136, -8.3) -> (31.2136, -10.4) projected
  line L10 (50.3552, -10.4) -> (43.9577, -10.4) projected
  line L11 (54, -5.3) -> (51.2306, -5.3) projected
  line L12 (51.2306, -5.3) -> (51.2306, -8.3) projected
  line L13 (51.2306, -8.3) -> (45.8, -8.3) projected
  line L14 (54, -5.3) -> (54, -13.6) projected
  line L15 (54, -13.6) -> (50.3552, -13.6) projected
  line L16 (50.3552, -10.4) -> (50.3552, -13.6) projected
  line L17 (3.6448, -13.6) -> (0, -13.6) projected
  line L18 (3.6448, -10.4) -> (3.6448, -13.6) projected
  line L19 (16.9577, -9.4) -> (16.9577, -10.4) projected
  line L20 (37.0423, -10.4) -> (31.2136, -10.4) projected
  line L21 (37.0423, -10.4) -> (37.0423, -9.4) projected
  line L22 (37.0423, -9.4) -> (43.9577, -9.4) projected
  line L23 (43.9577, -9.4) -> (43.9577, -10.4) projected
  line L24 (10.0423, -10.4) -> (3.6448, -10.4) projected
  line L25 (10.0423, -10.4) -> (10.0423, -9.4) projected
  line L26 (10.0423, -9.4) -> (16.9577, -9.4) projected
  point P0 (39.5, 16.2)
  dimension "d56" = 7
  dimension "d55" = 7
  dimension "d57" = 3.5
  constraints: 2 coincident, 2 tangent, 1 centre point, 3 other
  measures "d55" diameter of A0
  measures "d57" distance from line of L1 point (24.298, -3.5)
hole "Hole1" at (36, -19.7, 0) at (15.2017, -19.7, 0) direction (0, 0, 1) diameter 4 depth 6 counterbore diameter 5 counterbore depth 1
sketch "Sketch13" plane through (39.5, -16.2, 27.7) normal (1, 0, 0) x (0, 0, -1)
  line L0 (0, 0) -> (27.7, 0) projected
  line L1 (0, 0) -> (0, -13.6) projected
  line L2 (27.7, 0) -> (27.7, -13.6) projected
  circle A0 centre (3.5, -10) radius 3.5
  line L3 (13.3727, -10.4) -> (27.7, -10.4) projected
  circle A1 centre (17.2, -3.5) radius 3.5
  line L4 (27.7, -13.6) -> (0, -13.6) projected
  point P0 (27.7, 16.2)
  point P1 (3.541, -13.6)
  dimension "d65" = 7
  dimension "d67" = 3.5
  dimension "d68" = 7
  dimension "d69" = 10.5
  dimension "d70" = 3.5
  constraints: 2 centre point, 2 coincident
  measures "d65" diameter of A0
  measures "d67" distance from line of L1 A0.centre
  measures "d68" diameter of A1
  measures "d69" distance from line of L2 A1.centre
  measures "d70" distance from line of L0 A1.centre
hole "Hole2" at (39.5, -26.2, 24.2) at (39.5, -19.7, 10.5) direction (-1, 0, 0) diameter 4 depth 5 counterbore diameter 5 counterbore depth 1
sketch "Sketch14" plane through (-14.5, -21.5, 0) normal (-1, 0, 0) x (0, 0, 1)
  line L0 (27.7, 0) -> (0, 0) projected
  line L1 (27.7, 0) -> (27.7, -0.4) projected
  circle A0 centre (24.2, -4.15) radius 3.5
  point P0 (0, 21.5)
  dimension "d79" = 7
  dimension "d80" = 4.15
  constraints: 1 centre point, 1 coincident, 1 tangent
  measures "d79" diameter of A0
  measures "d80" distance from line of L0 A0.centre
hole "Hole3" at (-14.5, -25.65, 24.2) direction (1, 0, 0) diameter 4 depth 6 counterbore diameter 5 counterbore depth 1
sketch "Sketch15" plane through (4.1095, -16.2, 27.7) normal (0, 0, 1) x (1, 0, 0)
  line L0 (0, 0) -> (12.89, 0) projected
  line L1 (0, 0) -> (0, -5.3) projected
  line L2 (12.89, 0) -> (12.89, -13.6) projected
  line L3 (23.0079, 0) -> (35.3905, 0) projected
  line L4 (35.3905, 0) -> (35.3905, -13.6) projected
  circle A0 centre (31.8905, -3.5) radius 3.5
  line L5 (-11.5832, -13.4998) -> (-11.6095, -5.3)
  line L6 (-12.5595, -5.3) -> (-0.4375, -5.3) projected
  circle A1 centre (-8.3433, -10.35) radius 3.25
  line L7 (1.9951, -5.3) -> (1.9951, -5.7) projected
  line L8 (3.4961, -5.7) -> (16.1671, -5.7) projected
  line L9 (-18.6095, -5.3) -> (-18.6095, -13.6) projected
  line L10 (0, 0) -> (12.89, 0) projected
  line L11 (0, 0) -> (0, -5.3) projected
  line L12 (0, -5.3) -> (-18.6095, -5.3) projected
  line L13 (-18.6095, -5.3) -> (-18.6095, -13.6) projected
  line L14 (23.0079, 0) -> (23.0079, -13.6) projected
  line L15 (12.89, 0) -> (12.89, -13.6) projected
  line L16 (0, -5.3) -> (-18.6095, -5.3) projected
  line L17 (35.3905, 0) -> (35.3905, -13.6) projected
  line L18 (23.0079, 0) -> (35.3905, 0) projected
  line L19 (23.0079, 0) -> (23.0079, -13.6) projected
  line L20 (35.3905, -13.6) -> (23.0079, -13.6) projected
  line L21 (12.89, -13.6) -> (-18.6095, -13.6) projected
  line L22 (35.3905, -13.6) -> (23.0079, -13.6) projected
  line L23 (12.89, -13.6) -> (-18.6095, -13.6) projected
  point P0 (-4.1095, 16.2)
  point P1 (-9.3064, -5.3)
  point P2 (1.9951, -8.3)
  point P3 (11.1823, -5.7)
  point P4 (-3.8692, -5.3)
  point P5 (-10.4095, -5.3)
  point P6 (11.1823, -5.7)
  point P7 (16.2843, -5.7)
  dimension "d89" = 7
  dimension "d91" = 6.5
  constraints: 4 tangent, 2 centre point, 2 end point, 1 coincident, 1 point on line
  measures "d89" diameter of A0
  measures "d91" diameter of A1
hole "Hole4" at (-4.2338, -26.55, 27.7) at (36, -19.7, 27.7) direction (0, 0, -1) diameter 4 depth 5.2 counterbore diameter 5 counterbore depth 1
sketch "Sketch17" plane through (-21, -29.8, 14.3) normal (0, -1, 0) x (1, 0, 0)
  arc A0 (27.2086, -1.4674) -> (10.1448, -14.3) centre (20, -9.6433) ccw projected
  circle A1 centre (10, 0.7181) radius 3.5
  circle A2 centre (26.6771, 9.9) radius 3.5
  circle A3 centre (57, 0.7181) radius 3.5
  line L0 (57, 0.7181) -> (54.5694, -1.8003)
  line L1 (26.6771, 9.9) -> (29.3133, 7.5978)
  line L2 (10, 0.7181) -> (12.4306, -1.8003)
  line L3 (6.5, -14.3) -> (10.1448, -14.3) projected
  arc A4 (49.3884, 4.2041) -> (36.2919, 9.8389) centre (43.0585, 7.5289) ccw projected
  arc A5 (52.0289, 0.0273) -> (49.3884, 4.2041) centre (46.65, -0.45) ccw projected
  arc A6 (56.8552, -14.3) -> (52.0289, 0.0273) centre (47, -9.6433) ccw projected
  line L4 (56.8552, -14.3) -> (60.5, -14.3) projected
  line L5 (60.5, -14.3) -> (60.5, 13.4) projected
  line L6 (60.5, 13.4) -> (48.1174, 13.4) projected
  arc A7 (48.1174, 13.4) -> (37.9995, 13.4) centre (43.0585, 7.5289) ccw projected
  line L7 (37.9995, 13.4) -> (6.5, 13.4) projected
  line L8 (6.5, 13.4) -> (6.5, -14.3) projected
  arc A8 (29.092, 0.1172) -> (27.2086, -1.4674) centre (33.5, -7.0333) ccw projected
  arc A9 (36.2919, 9.8389) -> (29.092, 0.1172) centre (35.7557, 2.709) ccw projected
  point P0 (21, -14.3)
  dimension "d115" = 7
  dimension "d116" = 7
  dimension "d117" = 7
  dimension "d121" = 3.5
  dimension "d122" = 3.5
  dimension "d123" = 3.5
  constraints: 6 end point, 3 centre point, 3 coincident, 1 line through centre, 1 point on circle
  measures "d115" diameter of A1
  measures "d116" diameter of A2
  measures "d117" diameter of A3
  measures "d121" distance of L0.start L0.end
  measures "d122" distance of L1.start L1.end
  measures "d123" distance of L2.start L2.end
hole "Hole6" at (36, -29.8, 15.0181) at (-11, -29.8, 15.0181) at (5.6771, -29.8, 24.2) direction (0, 1, 0) diameter 4 depth 5 counterbore diameter 5 counterbore depth 1
sketch "Sketch18" plane through (-21, -18.8, 14.3) normal (0, -1, 0) x (1, 0, 0)
  circle A0 centre (43.0585, 7.5289) radius 1.25 projected
  circle A1 centre (43.0585, 7.5289) radius 1.45
  point P0 (21, -14.3)
  dimension "d131" = 0.2
  constraints: 1 centre point
  measures "d131" radial gap between concentric circles of A0 A1
extrude "Extrusion12" cut sketch "Sketch18" against normal blind 2 contours A0 | A1
sketch "Sketch19" plane through (-21, -21.9, 14.3) normal (0, -1, 0) x (1, 0, 0)
  circle A0 centre (35.7557, 2.709) radius 1.25 projected
  circle A1 centre (35.7557, 2.709) radius 1.45
  point P0 (21, -14.3)
  dimension "d134" = 0.2
  constraints: 1 centre point
  measures "d134" radial gap between concentric circles of A0 A1
extrude "Extrusion13" cut sketch "Sketch19" against normal blind 5.1 contours A0 | A1
sketch "Sketch20" plane through (-21, -24.5, 14.3) normal (0, -1, 0) x (1, 0, 0)
  circle A0 centre (33.5, -7.0333) radius 1.25 projected
  circle A1 centre (33.5, -7.0333) radius 1.45
  point P0 (21, -14.3)
  dimension "d137" = 0.2
  constraints: 1 centre point
  measures "d137" radial gap between concentric circles of A0 A1
extrude "Extrusion14" cut sketch "Sketch20" against normal blind 2.4 contours A0 | A1
sketch "Sketch21" plane through (-21, -19.2, 14.3) normal (0, -1, 0) x (1, 0, 0)
  point P0 (21, -14.3)
sketch "Sketch22" plane through (-21, -19.2, 14.3) normal (0, -1, 0) x (1, 0, 0)
  circle A0 centre (40.0468, 4.0664) radius 1.0564 projected
  circle A1 centre (40.0468, 4.0664) radius 2.25
  point P0 (21, -14.3)
  dimension "d146" = 4.5
  constraints: 1 centre point, 1 coincident
  measures "d146" diameter of A1
extrude "Extrusion15" cut sketch "Sketch22" against normal blind 2.4 contours A0 | A1
sketch "Sketch23" plane through (19.0468, -16.8, 18.3664) normal (0, -1, 0) x (1, 0, 0)
  point P0 (-19.0468, -18.3664)
sketch "Sketch24" plane through (19.0468, -16.8, 18.3664) normal (0, -1, 0) x (1, 0, 0)
  circle A0 centre (0, 0) radius 1.0564 projected
  circle A1 centre (0, 0) radius 1.25
  point P0 (-19.0468, -18.3664)
  dimension "d149" = 2.5
  constraints: 2 coincident, 1 centre point
  measures "d149" diameter of A1
extrude "Extrusion16" cut sketch "Sketch24" against normal blind 2.4 contours A0 | A1
sketch "Sketch25" plane through (-21, -26.6, 14.3) normal (0, -1, 0) x (1, 0, 0)
  circle A0 centre (53.2532, -4.9664) radius 1.0564 projected
  circle A1 centre (53.2532, -4.9664) radius 2.25
  point P0 (21, -14.3)
  dimension "d152" = 4.5
  constraints: 2 coincident, 1 centre point
  measures "d152" diameter of A1
hole "Hole7" at (32.2532, -26.6, 9.3336) direction (0, 1, 0) diameter 2.6 end through all counterbore diameter 4.5 counterbore depth 3.7
equation "\"d57\" = 0.5 * d56"
equation "\"d67\" = 0.5 * d65"
body "Solid1"
